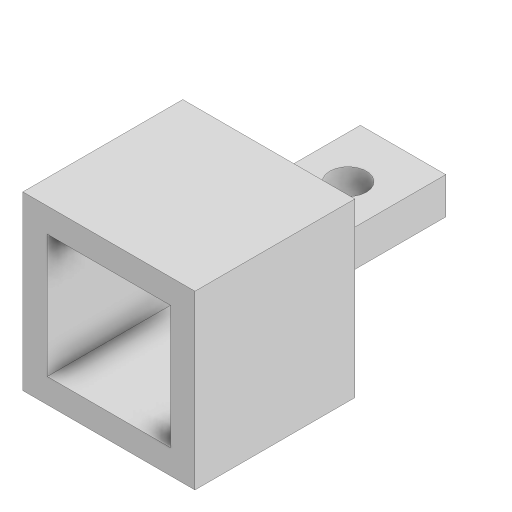
# Autodesk Inventor part: adapter_for_magnet
Saved by Autodesk Inventor 2024 (Build 280153000, 153)
## iProperties
Created: 2023-11-12
Part Number: adapter_for_magnet
Material: 一般
Document SubType Name: Modeling
Designer: moonshot
Density: 1 g/cm^3
Appearance: 既定
Author: moonshot
Autodesk Inventor part; units mm, degrees
ref_plane "YZ Plane" through (0, 0, 0) normal (1, 0, 0) x (0, 1, 0)
ref_plane "XZ Plane" through (0, 0, 0) normal (0, 1, 0) x (-1, 0, 0)
ref_plane "XY Plane" through (0, 0, 0) normal (0, 0, 1) x (1, 0, 0)
sketch "スケッチ1" plane through (0, 0, 0) normal (0, 0, 1) x (1, 0, 0)
  line L0 (-5.05, 5.05) -> (5.05, 5.05)
  line L1 (5.05, 5.05) -> (5.05, -5.05)
  line L2 (5.05, -5.05) -> (-5.05, -5.05)
  line L3 (-5.05, -5.05) -> (-5.05, 5.05)
  line L4 (0, -9.87) -> (0, 9.87) projected
  line L5 (-9.87, 0) -> (9.87, 0) projected
  line L6 (7.05, 7.05) -> (-7.05, 7.05)
  line L7 (-7.05, 7.05) -> (-7.05, -7.05)
  line L8 (-7.05, -7.05) -> (7.05, -7.05)
  line L9 (7.05, -7.05) -> (7.05, 7.05)
  point P0 (0, 0)
  dimension "d0" = 10.1
  dimension "d1" = 2
  dimension "d27" = 10.1
  constraints: 16 end point, 4 parallel, 2 perpendicular, 1 horizontal, 5 other
  measures "d0" distance of L0.start L0.end
  measures "d1" distance between parallel lines of L0 L6
  measures "d27" distance of L2.end L0.start
extrude "押し出し1" add sketch "スケッチ1" along normal mid plane 10.1 contours L3 L5 L7 L6 L4 L0 | L4 L6 L9 L5 L1 L0 | L3 L2 L4 L8 L7 L5 | L5 L9 L8 L4 L2 L1
sketch "スケッチ2" plane through (0, 0, -5.05) normal (0, 0, -1) x (-1, 0, 0)
  line L0 (-7.05, -7.05) -> (-7.05, 7.05) projected
  line L1 (7.05, 7.05) -> (-7.05, 7.05) projected
  line L2 (-7.05, -7.05) -> (7.05, -7.05) projected
  line L3 (7.05, -7.05) -> (7.05, 7.05) projected
  line L4 (7.05, 7.05) -> (-7.05, 7.05) projected
  line L5 (-7.05, 7.05) -> (-7.05, -7.05) projected
  line L6 (5.05, 5.05) -> (5.05, -5.05) projected
  line L7 (5.05, -5.05) -> (-5.05, -5.05) projected
  line L8 (-5.05, -5.05) -> (-5.05, 5.05) projected
  line L9 (-5.05, 5.05) -> (5.05, 5.05) projected
  line L10 (-7.05, 7.05) -> (7.05, 7.05) projected
  line L11 (-7.05, 7.05) -> (7.05, 7.05)
  line L12 (7.05, 7.05) -> (7.05, -7.05) projected
  line L13 (7.05, -7.05) -> (-7.05, -7.05)
  line L14 (9.87, 0) -> (-9.87, 0) projected
  line L15 (0, -10.0068) -> (0, 10.0068) projected
  line L16 (-7.05, 7.05) -> (-7.05, -7.05)
  line L17 (7.05, 7.05) -> (7.05, -7.05)
  point P0 (0, 0)
  constraints: 8 end point, 2 equal length, 1 perpendicular
extrude "押し出し2" add sketch "スケッチ2" along normal blind 3
sketch "スケッチ4" plane through (0, 0, -8.05) normal (0, 0, -1) x (-1, 0, 0)
  line L0 (3.5, 1.5) -> (-3.5, 1.5)
  line L1 (-3.5, 1.5) -> (-3.5, -1.5)
  line L2 (-3.5, -1.5) -> (3.5, -1.5)
  line L3 (3.5, -1.5) -> (3.5, 1.5)
  line L4 (9.87, 0) -> (-9.87, 0) projected
  line L5 (0, -9.87) -> (0, 9.87) projected
  point P0 (0, 0)
  dimension "d19" = 3
  dimension "d20" = 7
  constraints: 8 end point, 2 parallel, 1 horizontal, 1 perpendicular, 2 other
  measures "d19" distance between parallel lines of L0 L2
  measures "d20" distance of L1.end L2.end
extrude "押し出し4" add sketch "スケッチ4" along normal blind 11
sketch "スケッチ5" plane through (-3.5, 1.5, -8.05) normal (0, 1, 0) x (1, 0, 0)
  circle A0 centre (3.5, 6.5) radius 1.5
  line L0 (-3.55, 0) -> (10.55, 0) projected
  line L1 (3.5, 15.82) -> (3.5, -17.92) projected
  point P0 (3.5, -8.05)
  dimension "d23" = 3
  dimension "d24" = 6.5
  constraints: 1 centre point, 1 point on line
  measures "d23" diameter of A0
  measures "d24" distance from line of L0 A0.centre
extrude "押し出し5" cut sketch "スケッチ5" against normal up to surface (3 mm away)
